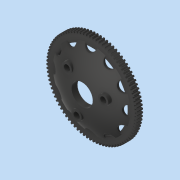
# Autodesk Inventor part: SpurGearLarge
Saved by Autodesk Inventor 2017 (Build 210142000, 142)
## iProperties
Created: 2016-11-06
Part Number: SpurGearLarge
Material: ABS Plastic
Document SubType Name: Modeling
Designer: techn
Density: 1.06 g/cm^3
Appearance: Smooth - Black
Author: techn
Autodesk Inventor part; units mm, degrees
ref_plane "YZ Plane" through (0, 0, 0) normal (1, 0, 0) x (0, 1, 0)
ref_plane "XZ Plane" through (0, 0, 0) normal (0, 1, 0) x (-1, 0, 0)
ref_plane "XY Plane" through (0, 0, 0) normal (0, 0, 1) x (1, 0, 0)
sketch "Sketch5" plane through (0, 0, 0) normal (0, 0, 1) x (1, 0, 0)
  circle A0 centre (0, 0) radius 22.86
  circle A1 centre (0, 0) radius 18.415
  dimension "d23" = 45.72
  dimension "d24" = 36.83
  constraints: 2 centre point, 2 coincident
  measures "d23" diameter of A0
  measures "d24" diameter of A1
extrude "Extrusion5" add sketch "Sketch5" along normal blind 3.175
sketch "Sketch6" plane through (0, 0, 0) normal (1, 0, 0) x (0, 1, 0)
  line L0 (22.86, 3.175) -> (-22.86, 3.175)
  line L1 (-22.86, 0) -> (22.86, 0)
  line L2 (22.86, 3.175) -> (-22.86, 3.175)
  line L3 (0, 3.175) -> (5.461, 3.175)
  line L4 (5.461, 3.175) -> (5.461, 7.9375)
  line L5 (22.86, 3.175) -> (19.685, 3.175)
  arc A0 (19.685, 3.175) -> (5.461, 7.9375) centre (0.085817, -31.738803) ccw
  line L6 (0, 3.175) -> (0, 13.966627)
  line L7 (-18.415, 3.175) -> (18.415, 3.175)
  line L8 (19.685, 3.175) -> (18.415, 3.175)
  arc A1 (18.415, 3.175) -> (5.461, 5.715) centre (1.432553, -49.132779) ccw
  point P0 (0, 0)
  dimension "d27" = 5.461
  dimension "d28" = 4.7625
  dimension "d29" = 3.175
  dimension "d36" = 2.54
  constraints: 10 end point, 4 point on circle, 3 point on line, 2 centre point, 1 horizontal, 1 midpoint, 1 perpendicular, 1 vertical
  measures "d27" distance of L3.start L3.end
  measures "d28" distance of L3.end L4.end
  measures "d29" distance of L0.start L5.end
  measures "d36" distance of L3.end A1.end
revolve "Revolution3" add sketch "Sketch6" angle 360 about axis through (0, 0, 3.175) along (0, 0, 1) contours L0 A1 L4 A0
sketch "Sketch8" plane through (0, 0, 3.175) normal (0, 0, 1) x (1, 0, 0)
  circle A0 centre (0, 0) radius 19.685
  circle A1 centre (0, 19.685) radius 2.8575
  circle A2 centre (-9.8425, 17.04771) radius 2.8575
  circle A3 centre (-17.04771, 9.8425) radius 2.8575
  circle A4 centre (-19.685, 0) radius 2.8575
  circle A5 centre (-17.04771, -9.8425) radius 2.8575
  circle A6 centre (-9.8425, -17.04771) radius 2.8575
  circle A7 centre (0, -19.685) radius 2.8575
  circle A8 centre (9.8425, -17.04771) radius 2.8575
  circle A9 centre (17.04771, -9.8425) radius 2.8575
  circle A10 centre (19.685, 0) radius 2.8575
  circle A11 centre (17.04771, 9.8425) radius 2.8575
  circle A12 centre (9.8425, 17.04771) radius 2.8575
  dimension "d38" = 5.715
  dimension "d41" = 360
  constraints: 12 centre point, 1 vertical alignment, 26 other
  measures "d38" diameter of A1
extrude "Extrusion6" cut sketch "Sketch8" along normal blind 3.175 contours A0 A10 | A0 A10 | A11 A0 | A0 A11 | A9 A0 | A0 A9 | A12 A0 | A0 A12 | A8 A0 | A0 A8 | A1 A0 | A0 A1 | A7 A0 | A0 A7 | A2 A0 | A0 A2 | A6 A0 | A0 A6 | A3 A0 | A0 A3 | A5 A0 | A0 A5 | A4 A0 | A0 A4
ref_plane "Work Plane1" through (0, 0, 7.9375) normal (0, 0, 1) x (1, 0, 0)
sketch "Sketch9" plane through (0, 0, 7.9375) normal (0, 0, 1) x (1, 0, 0)
  line L0 (0, 0) -> (12.7, 0) construction
  circle A0 centre (-7.77713, 7.77713) radius 1.5875
  circle A1 centre (-7.77713, 7.77713) radius 2.54
  circle A2 centre (-2.846627, -10.623757) radius 2.54
  circle A3 centre (-2.846627, -10.623757) radius 1.5875
  circle A4 centre (10.623757, 2.846627) radius 2.54
  circle A5 centre (10.623757, 2.846627) radius 1.5875
  dimension "d48" = 3.175
  dimension "d49" = 5.08
  dimension "d52" = 360
  dimension "d58" = 19.05
  constraints: 6 centre point, 3 coincident, 2 end point, 1 horizontal, 13 other
  measures "d48" diameter of A0
  measures "d49" diameter of A1
  measures "d58" distance of A4.centre A0.centre
extrude "Extrusion7" add sketch "Sketch9" against normal blind 2.286
extrude "Extrusion8" cut sketch "Sketch9" against normal through all contours A0 | A3 | A5
sketch "Sketch10" plane through (0, 0, 3.175) normal (0, 0, 1) x (1, 0, 0)
  circle A0 centre (0, 0) radius 21.8948
  line L0 (0.3683, 21.891702) -> (0.3683, 22.399702)
  line L1 (0.3683, 22.399702) -> (0.272875, 22.86)
  line L2 (0.272875, 22.86) -> (-0.272875, 22.86)
  line L3 (-0.272875, 22.86) -> (-0.3683, 22.399702)
  line L4 (-0.3683, 22.399702) -> (-0.3683, 21.891702)
  line L5 (-0.3683, 21.891702) -> (0.3683, 21.891702)
  line L6 (-1.983652, 22.314736) -> (-1.946996, 21.80806)
  line L7 (-1.92169, 22.780719) -> (-1.983652, 22.314736)
  line L8 (-1.377363, 22.820099) -> (-1.92169, 22.780719)
  line L9 (-1.248972, 22.367887) -> (-1.377363, 22.820099)
  line L10 (-1.212316, 21.861211) -> (-1.248972, 22.367887)
  line L11 (-1.946996, 21.80806) -> (-1.212316, 21.861211)
  line L12 (-3.588662, 22.11343) -> (-3.515541, 21.61072)
  line L13 (-3.560486, 22.58267) -> (-3.588662, 22.11343)
  line L14 (-3.02042, 22.661225) -> (-3.560486, 22.58267)
  line L15 (-2.859733, 22.219456) -> (-3.02042, 22.661225)
  line L16 (-2.786612, 21.716746) -> (-2.859733, 22.219456)
  line L17 (-3.515541, 21.61072) -> (-2.786612, 21.716746)
  line L18 (-5.174963, 21.796836) -> (-5.065758, 21.300713)
  line L19 (-5.180719, 22.266886) -> (-5.174963, 21.796836)
  line L20 (-4.647729, 22.384206) -> (-5.180719, 22.266886)
  line L21 (-4.455584, 21.955183) -> (-4.647729, 22.384206)
  line L22 (-4.346379, 21.45906) -> (-4.455584, 21.955183)
  line L23 (-5.065758, 21.300713) -> (-4.346379, 21.45906)
  line L24 (-6.734284, 21.366603) -> (-6.589565, 20.879653)
  line L25 (-6.773943, 21.835012) -> (-6.734284, 21.366603)
  line L26 (-6.250808, 21.990486) -> (-6.773943, 21.835012)
  line L27 (-6.028207, 21.576446) -> (-6.250808, 21.990486)
  line L28 (-5.883487, 21.089496) -> (-6.028207, 21.576446)
  line L29 (-6.589565, 20.879653) -> (-5.883487, 21.089496)
  line L30 (-8.258495, 20.824974) -> (-8.079016, 20.349736)
  line L31 (-8.33185, 21.289301) -> (-8.258495, 20.824974)
  line L32 (-7.821297, 21.482117) -> (-8.33185, 21.289301)
  line L33 (-7.5694, 21.085219) -> (-7.821297, 21.482117)
  line L34 (-7.389921, 20.609981) -> (-7.5694, 21.085219)
  line L35 (-8.079016, 20.349736) -> (-7.389921, 20.609981)
  line L36 (-9.739651, 20.174774) -> (-9.526347, 19.713726)
  line L37 (-9.846319, 20.632597) -> (-9.739651, 20.174774)
  line L38 (-9.351011, 20.861751) -> (-9.846319, 20.632597)
  line L39 (-9.071131, 20.484064) -> (-9.351011, 20.861751)
  line L40 (-8.857827, 20.023016) -> (-9.071131, 20.484064)
  line L41 (-9.526347, 19.713726) -> (-8.857827, 20.023016)
  line L42 (-11.170028, 19.419392) -> (-10.924012, 18.974937)
  line L43 (-11.309454, 19.868324) -> (-11.170028, 19.419392)
  line L44 (-10.831972, 20.132621) -> (-11.309454, 19.868324)
  line L45 (-10.525569, 19.776115) -> (-10.831972, 20.132621)
  line L46 (-10.279553, 19.33166) -> (-10.525569, 19.776115)
  line L47 (-10.924012, 18.974937) -> (-10.279553, 19.33166)
  line L48 (-12.54217, 18.562766) -> (-12.264725, 18.137221)
  line L49 (-12.713627, 19.000467) -> (-12.54217, 18.562766)
  line L50 (-12.25646, 19.29853) -> (-12.713627, 19.000467)
  line L51 (-11.925131, 18.965061) -> (-12.25646, 19.29853)
  line L52 (-11.647685, 18.539517) -> (-11.925131, 18.965061)
  line L53 (-12.264725, 18.137221) -> (-11.647685, 18.539517)
  line L54 (-13.848923, 17.609362) -> (-13.541495, 17.204947)
  line L55 (-14.051516, 18.033551) -> (-13.848923, 17.609362)
  line L56 (-13.617049, 18.363824) -> (-14.051516, 18.033551)
  line L57 (-13.262521, 18.055133) -> (-13.617049, 18.363824)
  line L58 (-12.955093, 17.650718) -> (-13.262521, 18.055133)
  line L59 (-13.541495, 17.204947) -> (-12.955093, 17.650718)
  line L60 (-15.083474, 16.564151) -> (-14.747666, 16.182973)
  line L61 (-15.316148, 16.972616) -> (-15.083474, 16.564151)
  line L62 (-14.906645, 17.333378) -> (-15.316148, 16.972616)
  line L63 (-14.530767, 17.051074) -> (-14.906645, 17.333378)
  line L64 (-14.194958, 16.669896) -> (-14.530767, 17.051074)
  line L65 (-14.747666, 16.182973) -> (-14.194958, 16.669896)
  line L66 (-16.239387, 15.432583) -> (-15.876949, 15.07663)
  line L67 (-16.500928, 15.823193) -> (-16.239387, 15.432583)
  line L68 (-16.118524, 16.212564) -> (-16.500928, 15.823193)
  line L69 (-15.723256, 15.958118) -> (-16.118524, 16.212564)
  line L70 (-15.360817, 15.602165) -> (-15.723256, 15.958118)
  line L71 (-15.876949, 15.07663) -> (-15.360817, 15.602165)
  line L72 (-17.310635, 14.220556) -> (-16.923457, 13.891683)
  line L73 (-17.59968, 14.591276) -> (-17.310635, 14.220556)
  line L74 (-17.246369, 15.007225) -> (-17.59968, 14.591276)
  line L75 (-16.833771, 14.781964) -> (-17.246369, 15.007225)
  line L76 (-16.446592, 14.453092) -> (-16.833771, 14.781964)
  line L77 (-16.923457, 13.891683) -> (-16.446592, 14.453092)
  line L78 (-18.291634, 12.934389) -> (-17.881734, 12.634312)
  line L79 (-18.606675, 13.283286) -> (-18.291634, 12.934389)
  line L80 (-18.2843, 13.723646) -> (-18.606675, 13.283286)
  line L81 (-17.856522, 13.528744) -> (-18.2843, 13.723646)
  line L82 (-17.446623, 13.228667) -> (-17.856522, 13.528744)
  line L83 (-17.881734, 12.634312) -> (-17.446623, 13.228667)
  line L84 (-19.177268, 11.580789) -> (-18.746784, 11.311072)
  line L85 (-19.516664, 11.906044) -> (-19.177268, 11.580789)
  line L86 (-19.226904, 12.368517) -> (-19.516664, 11.906044)
  line L87 (-18.786178, 12.204991) -> (-19.226904, 12.368517)
  line L88 (-18.355694, 11.935274) -> (-18.786178, 12.204991)
  line L89 (-18.746784, 11.311072) -> (-18.355694, 11.935274)
  line L90 (-19.962921, 10.166812) -> (-19.514097, 9.928861)
  line L91 (-20.324902, 10.466729) -> (-19.962921, 10.166812)
  line L92 (-20.069269, 10.948905) -> (-20.324902, 10.466729)
  line L93 (-19.617892, 10.817607) -> (-20.069269, 10.948905)
  line L94 (-19.169068, 10.579656) -> (-19.617892, 10.817607)
  line L95 (-19.514097, 9.928861) -> (-19.169068, 10.579656)
  line L96 (-20.644497, 8.69983) -> (-20.179673, 8.494885)
  line L97 (-21.027175, 8.972845) -> (-20.644497, 8.69983)
  line L98 (-20.807001, 9.47221) -> (-21.027175, 8.972845)
  line L99 (-20.347327, 9.373825) -> (-20.807001, 9.47221)
  line L100 (-19.882503, 9.16888) -> (-20.347327, 9.373825)
  line L101 (-20.179673, 8.494885) -> (-19.882503, 9.16888)
  line L102 (-21.218442, 7.187491) -> (-20.740041, 7.016621)
  line L103 (-21.619823, 7.432181) -> (-21.218442, 7.187491)
  line L104 (-21.436255, 7.946132) -> (-21.619823, 7.432181)
  line L105 (-20.97068, 7.881172) -> (-21.436255, 7.946132)
  line L106 (-20.492279, 7.710302) -> (-20.97068, 7.881172)
  line L107 (-20.740041, 7.016621) -> (-20.492279, 7.710302)
  line L108 (-21.681764, 5.63768) -> (-21.19228, 5.501775)
  line L109 (-22.099755, 5.852769) -> (-21.681764, 5.63768)
  line L110 (-21.953751, 6.378626) -> (-22.099755, 5.852769)
  line L111 (-21.484702, 6.347431) -> (-21.953751, 6.378626)
  line L112 (-20.995219, 6.211526) -> (-21.484702, 6.347431)
  line L113 (-21.19228, 5.501775) -> (-20.995219, 6.211526)
  line L114 (-22.032046, 4.058476) -> (-21.534032, 3.958246)
  line L115 (-22.464468, 4.242844) -> (-22.032046, 4.058476)
  line L116 (-22.35679, 4.777865) -> (-22.464468, 4.242844)
  line L117 (-21.886713, 4.780596) -> (-22.35679, 4.777865)
  line L118 (-21.388699, 4.680366) -> (-21.886713, 4.780596)
  line L119 (-21.534032, 3.958246) -> (-21.388699, 4.680366)
  line L120 (-22.267465, 2.458114) -> (-21.763516, 2.39408)
  line L121 (-22.712063, 2.610798) -> (-22.267465, 2.458114)
  line L122 (-22.643271, 3.152195) -> (-22.712063, 2.610798)
  line L123 (-22.174616, 3.188838) -> (-22.643271, 3.152195)
  line L124 (-21.670668, 3.124805) -> (-22.174616, 3.188838)
  line L125 (-21.763516, 2.39408) -> (-21.670668, 3.124805)
  line L126 (-22.38679, 0.844936) -> (-21.879535, 0.817433)
  line L127 (-22.841247, 0.965141) -> (-22.38679, 0.844936)
  line L128 (-22.811701, 1.51009) -> (-22.841247, 0.965141)
  line L129 (-22.346912, 1.580455) -> (-22.811701, 1.51009)
  line L130 (-21.839657, 1.552953) -> (-22.346912, 1.580455)
  line L131 (-21.879535, 0.817433) -> (-21.839657, 1.552953)
  line L132 (-22.389402, -0.772648) -> (-21.881485, -0.763476)
  line L133 (-22.851348, -0.685548) -> (-22.389402, -0.772648)
  line L134 (-22.861201, -0.139888) -> (-22.851348, -0.685548)
  line L135 (-22.402701, -0.036168) -> (-22.861201, -0.139888)
  line L136 (-21.894783, -0.026996) -> (-22.402701, -0.036168)
  line L137 (-21.881485, -0.763476) -> (-21.894783, -0.026996)
  line L138 (-22.275285, -2.386202) -> (-21.769354, -2.340405)
  line L139 (-22.742312, -2.332663) -> (-22.275285, -2.386202)
  line L140 (-22.791513, -1.789136) -> (-22.742312, -2.332663)
  line L141 (-22.341692, -1.652602) -> (-22.791513, -1.789136)
  line L142 (-21.835761, -1.606804) -> (-22.341692, -1.652602)
  line L143 (-21.769354, -2.340405) -> (-21.835761, -1.606804)
  line L144 (-22.045036, -3.987317) -> (-21.543728, -3.905131)
  line L145 (-22.514708, -3.967616) -> (-22.045036, -3.987317)
  line L146 (-22.603001, -3.429056) -> (-22.514708, -3.967616)
  line L147 (-22.164204, -3.26042) -> (-22.603001, -3.429056)
  line L148 (-21.662897, -3.178235) -> (-22.164204, -3.26042)
  line L149 (-21.543728, -3.905131) -> (-21.662897, -3.178235)
  line L150 (-21.699854, -5.567643) -> (-21.205783, -5.449499)
  line L151 (-22.169723, -5.581885) -> (-21.699854, -5.567643)
  line L152 (-22.296647, -5.0511) -> (-22.169723, -5.581885)
  line L153 (-21.871163, -4.85124) -> (-22.296647, -5.0511)
  line L154 (-21.377092, -4.733096) -> (-21.871163, -4.85124)
  line L155 (-21.205783, -5.449499) -> (-21.377092, -4.733096)
  line L156 (-21.241539, -7.118942) -> (-20.757281, -6.965455)
  line L157 (-21.709156, -7.167051) -> (-21.241539, -7.118942)
  line L158 (-21.874048, -6.646808) -> (-21.709156, -7.167051)
  line L159 (-21.464095, -6.416768) -> (-21.874048, -6.646808)
  line L160 (-20.979837, -6.263281) -> (-21.464095, -6.416768)
  line L161 (-20.757281, -6.965455) -> (-20.979837, -6.263281)
  line L162 (-20.67248, -8.633127) -> (-20.20056, -8.445096)
  line L163 (-21.135406, -8.714852) -> (-20.67248, -8.633127)
  line L164 (-21.337409, -8.207864) -> (-21.135406, -8.714852)
  line L165 (-20.945124, -7.948842) -> (-21.337409, -8.207864)
  line L166 (-20.473204, -7.760812) -> (-20.945124, -7.948842)
  line L167 (-20.20056, -8.445096) -> (-20.473204, -7.760812)
  line L168 (-19.995645, -10.102302) -> (-19.538522, -9.880709)
  line L169 (-20.451467, -10.217218) -> (-19.995645, -10.102302)
  line L170 (-20.689526, -9.726128) -> (-20.451467, -10.217218)
  line L171 (-20.316954, -9.439475) -> (-20.689526, -9.726128)
  line L172 (-19.859832, -9.217882) -> (-20.316954, -9.439475)
  line L173 (-19.538522, -9.880709) -> (-19.859832, -9.217882)
  line L174 (-19.214561, -11.518808) -> (-18.77462, -11.264808)
  line L175 (-19.660903, -11.666316) -> (-19.214561, -11.518808)
  line L176 (-19.933778, -11.193684) -> (-19.660903, -11.666316)
  line L177 (-19.582861, -10.880894) -> (-19.933778, -11.193684)
  line L178 (-19.14292, -10.626894) -> (-19.582861, -10.880894)
  line L179 (-18.77462, -11.264808) -> (-19.14292, -10.626894)
  line L180 (-18.333302, -12.875261) -> (-17.912836, -12.590178)
  line L181 (-18.767837, -13.054592) -> (-18.333302, -12.875261)
  line L182 (-19.074104, -12.602881) -> (-18.767837, -13.054592)
  line L183 (-18.746672, -12.265585) -> (-19.074104, -12.602881)
  line L184 (-18.326206, -11.980502) -> (-18.746672, -12.265585)
  line L185 (-17.912836, -12.590178) -> (-18.326206, -11.980502)
  line L186 (-17.356461, -14.164588) -> (-16.957662, -13.849908)
  line L187 (-17.776923, -14.374806) -> (-17.356461, -14.164588)
  line L188 (-18.114987, -13.946373) -> (-17.776923, -14.374806)
  line L189 (-17.812747, -13.586329) -> (-18.114987, -13.946373)
  line L190 (-17.413948, -13.27165) -> (-17.812747, -13.586329)
  line L191 (-16.957662, -13.849908) -> (-17.413948, -13.27165)
  line L192 (-16.289132, -15.380068) -> (-15.914079, -15.037432)
  line L193 (-16.693329, -15.620077) -> (-16.289132, -15.380068)
  line L194 (-17.061426, -15.217155) -> (-16.693329, -15.620077)
  line L195 (-16.785954, -14.836241) -> (-17.061426, -15.217155)
  line L196 (-16.410901, -14.493605) -> (-16.785954, -14.836241)
  line L197 (-15.914079, -15.037432) -> (-16.410901, -14.493605)
  line L198 (-15.136879, -16.515362) -> (-14.787528, -16.146557)
  line L199 (-15.522704, -16.783913) -> (-15.136879, -16.515362)
  line L200 (-15.918915, -16.408601) -> (-15.522704, -16.783913)
  line L201 (-15.671647, -16.008803) -> (-15.918915, -16.408601)
  line L202 (-15.322296, -15.639997) -> (-15.671647, -16.008803)
  line L203 (-14.787528, -16.146557) -> (-15.322296, -15.639997)
  line L204 (-13.905709, -17.564554) -> (-13.583881, -17.171501)
  line L205 (-14.27115, -17.860244) -> (-13.905709, -17.564554)
  line L206 (-14.693411, -17.514501) -> (-14.27115, -17.860244)
  line L207 (-14.475636, -17.097903) -> (-14.693411, -17.514501)
  line L208 (-14.153807, -16.70485) -> (-14.475636, -17.097903)
  line L209 (-13.583881, -17.171501) -> (-14.153807, -16.70485)
  line L210 (-12.602041, -18.522172) -> (-12.309414, -18.106921)
  line L211 (-12.945194, -18.843461) -> (-12.602041, -18.522172)
  line L212 (-13.391301, -18.529088) -> (-12.945194, -18.843461)
  line L213 (-13.204155, -18.097862) -> (-13.391301, -18.529088)
  line L214 (-12.911527, -17.682611) -> (-13.204155, -18.097862)
  line L215 (-12.309414, -18.106921) -> (-12.911527, -17.682611)
  line L216 (-11.232672, -19.383224) -> (-10.970771, -18.947941)
  line L217 (-11.551747, -19.728437) -> (-11.232672, -19.383224)
  line L218 (-12.019376, -19.447073) -> (-11.551747, -19.728437)
  line L219 (-11.863833, -19.003467) -> (-12.019376, -19.447073)
  line L220 (-11.601932, -18.568184) -> (-11.863833, -19.003467)
  line L221 (-10.970771, -18.947941) -> (-11.601932, -18.568184)
  line L222 (-9.804741, -20.143221) -> (-9.574932, -19.690174)
  line L223 (-10.098074, -20.510557) -> (-9.804741, -20.143221)
  line L224 (-10.584787, -20.263671) -> (-10.098074, -20.510557)
  line L225 (-10.46166, -19.809997) -> (-10.584787, -20.263671)
  line L226 (-10.23185, -19.35695) -> (-10.46166, -19.809997)
  line L227 (-9.574932, -19.690174) -> (-10.23185, -19.35695)
  line L228 (-8.325693, -20.7982) -> (-8.129173, -20.329752)
  line L229 (-8.591755, -21.185745) -> (-8.325693, -20.7982)
  line L230 (-9.095014, -20.974622) -> (-8.591755, -21.185745)
  line L231 (-9.004943, -20.513247) -> (-9.095014, -20.974622)
  line L232 (-8.808424, -20.044798) -> (-9.004943, -20.513247)
  line L233 (-8.129173, -20.329752) -> (-8.808424, -20.044798)
  line L234 (-6.803239, -21.344748) -> (-6.641033, -20.86334)
  line L235 (-7.040642, -21.750481) -> (-6.803239, -21.344748)
  line L236 (-7.557824, -21.576222) -> (-7.040642, -21.750481)
  line L237 (-7.50128, -21.10955) -> (-7.557824, -21.576222)
  line L238 (-7.339075, -20.628142) -> (-7.50128, -21.10955)
  line L239 (-6.641033, -20.86334) -> (-7.339075, -20.628142)
  line L240 (-5.245315, -21.780013) -> (-5.11827, -21.288156)
  line L241 (-5.452823, -22.201819) -> (-5.245315, -21.780013)
  line L242 (-5.98123, -22.065334) -> (-5.452823, -22.201819)
  line L243 (-5.958508, -21.595798) -> (-5.98123, -22.065334)
  line L244 (-5.831463, -21.103941) -> (-5.958508, -21.595798)
  line L245 (-5.11827, -21.288156) -> (-5.831463, -21.103941)
  line L246 (-3.660045, -22.101728) -> (-3.568822, -21.601985)
  line L247 (-3.836576, -22.537408) -> (-3.660045, -22.101728)
  line L248 (-4.373454, -22.439407) -> (-3.836576, -22.537408)
  line L249 (-4.384671, -21.969455) -> (-4.373454, -22.439407)
  line L250 (-4.293449, -21.469713) -> (-4.384671, -21.969455)
  line L251 (-3.568822, -21.601985) -> (-4.293449, -21.469713)
  line L252 (-2.055693, -22.308214) -> (-2.000768, -21.803192)
  line L253 (-2.200326, -22.755497) -> (-2.055693, -22.308214)
  line L254 (-2.742876, -22.696491) -> (-2.200326, -22.755497)
  line L255 (-2.787975, -22.228574) -> (-2.742876, -22.696491)
  line L256 (-2.73305, -21.723552) -> (-2.787975, -22.228574)
  line L257 (-2.000768, -21.803192) -> (-2.73305, -21.723552)
  line L258 (-0.440623, -22.398396) -> (-0.422283, -21.890727)
  line L259 (-0.552604, -22.854949) -> (-0.440623, -22.398396)
  line L260 (-1.097998, -22.835246) -> (-0.552604, -22.854949)
  line L261 (-1.176743, -22.371803) -> (-1.097998, -22.835246)
  line L262 (-1.158403, -21.864134) -> (-1.176743, -22.371803)
  line L263 (-0.422283, -21.890727) -> (-1.158403, -21.864134)
  line L264 (1.176743, -22.371803) -> (1.158403, -21.864134)
  line L265 (1.097998, -22.835246) -> (1.176743, -22.371803)
  line L266 (0.552604, -22.854949) -> (1.097998, -22.835246)
  line L267 (0.440623, -22.398396) -> (0.552604, -22.854949)
  line L268 (0.422283, -21.890727) -> (0.440623, -22.398396)
  line L269 (1.158403, -21.864134) -> (0.422283, -21.890727)
  line L270 (2.787975, -22.228574) -> (2.73305, -21.723552)
  line L271 (2.742876, -22.696491) -> (2.787975, -22.228574)
  line L272 (2.200326, -22.755497) -> (2.742876, -22.696491)
  line L273 (2.055693, -22.308214) -> (2.200326, -22.755497)
  line L274 (2.000768, -21.803192) -> (2.055693, -22.308214)
  line L275 (2.73305, -21.723552) -> (2.000768, -21.803192)
  line L276 (4.384671, -21.969455) -> (4.293449, -21.469713)
  line L277 (4.373454, -22.439407) -> (4.384671, -21.969455)
  line L278 (3.836576, -22.537408) -> (4.373454, -22.439407)
  line L279 (3.660045, -22.101728) -> (3.836576, -22.537408)
  line L280 (3.568822, -21.601985) -> (3.660045, -22.101728)
  line L281 (4.293449, -21.469713) -> (3.568822, -21.601985)
  line L282 (5.958508, -21.595798) -> (5.831463, -21.103941)
  line L283 (5.98123, -22.065334) -> (5.958508, -21.595798)
  line L284 (5.452823, -22.201819) -> (5.98123, -22.065334)
  line L285 (5.245315, -21.780013) -> (5.452823, -22.201819)
  line L286 (5.11827, -21.288156) -> (5.245315, -21.780013)
  line L287 (5.831463, -21.103941) -> (5.11827, -21.288156)
  line L288 (7.50128, -21.10955) -> (7.339075, -20.628142)
  line L289 (7.557824, -21.576222) -> (7.50128, -21.10955)
  line L290 (7.040642, -21.750481) -> (7.557824, -21.576222)
  line L291 (6.803239, -21.344748) -> (7.040642, -21.750481)
  line L292 (6.641033, -20.86334) -> (6.803239, -21.344748)
  line L293 (7.339075, -20.628142) -> (6.641033, -20.86334)
  line L294 (9.004943, -20.513247) -> (8.808424, -20.044798)
  line L295 (9.095014, -20.974622) -> (9.004943, -20.513247)
  line L296 (8.591755, -21.185745) -> (9.095014, -20.974622)
  line L297 (8.325693, -20.7982) -> (8.591755, -21.185745)
  line L298 (8.129173, -20.329752) -> (8.325693, -20.7982)
  line L299 (8.808424, -20.044798) -> (8.129173, -20.329752)
  line L300 (10.46166, -19.809997) -> (10.23185, -19.35695)
  line L301 (10.584787, -20.263671) -> (10.46166, -19.809997)
  line L302 (10.098074, -20.510557) -> (10.584787, -20.263671)
  line L303 (9.804741, -20.143221) -> (10.098074, -20.510557)
  line L304 (9.574932, -19.690174) -> (9.804741, -20.143221)
  line L305 (10.23185, -19.35695) -> (9.574932, -19.690174)
  line L306 (11.863833, -19.003467) -> (11.601932, -18.568184)
  line L307 (12.019376, -19.447073) -> (11.863833, -19.003467)
  line L308 (11.551747, -19.728437) -> (12.019376, -19.447073)
  line L309 (11.232672, -19.383224) -> (11.551747, -19.728437)
  line L310 (10.970771, -18.947941) -> (11.232672, -19.383224)
  line L311 (11.601932, -18.568184) -> (10.970771, -18.947941)
  line L312 (13.204155, -18.097862) -> (12.911527, -17.682611)
  line L313 (13.391301, -18.529088) -> (13.204155, -18.097862)
  line L314 (12.945194, -18.843461) -> (13.391301, -18.529088)
  line L315 (12.602041, -18.522172) -> (12.945194, -18.843461)
  line L316 (12.309414, -18.106921) -> (12.602041, -18.522172)
  line L317 (12.911527, -17.682611) -> (12.309414, -18.106921)
  line L318 (14.475636, -17.097903) -> (14.153807, -16.70485)
  line L319 (14.693411, -17.514501) -> (14.475636, -17.097903)
  line L320 (14.27115, -17.860244) -> (14.693411, -17.514501)
  line L321 (13.905709, -17.564554) -> (14.27115, -17.860244)
  line L322 (13.583881, -17.171501) -> (13.905709, -17.564554)
  line L323 (14.153807, -16.70485) -> (13.583881, -17.171501)
  line L324 (15.671647, -16.008803) -> (15.322296, -15.639997)
  line L325 (15.918915, -16.408601) -> (15.671647, -16.008803)
  line L326 (15.522704, -16.783913) -> (15.918915, -16.408601)
  line L327 (15.136879, -16.515362) -> (15.522704, -16.783913)
  line L328 (14.787528, -16.146557) -> (15.136879, -16.515362)
  line L329 (15.322296, -15.639997) -> (14.787528, -16.146557)
  line L330 (16.785954, -14.836241) -> (16.410901, -14.493605)
  line L331 (17.061426, -15.217155) -> (16.785954, -14.836241)
  line L332 (16.693329, -15.620077) -> (17.061426, -15.217155)
  line L333 (16.289132, -15.380068) -> (16.693329, -15.620077)
  line L334 (15.914079, -15.037432) -> (16.289132, -15.380068)
  line L335 (16.410901, -14.493605) -> (15.914079, -15.037432)
  line L336 (17.812747, -13.586329) -> (17.413948, -13.27165)
  line L337 (18.114987, -13.946373) -> (17.812747, -13.586329)
  line L338 (17.776923, -14.374806) -> (18.114987, -13.946373)
  line L339 (17.356461, -14.164588) -> (17.776923, -14.374806)
  line L340 (16.957662, -13.849908) -> (17.356461, -14.164588)
  line L341 (17.413948, -13.27165) -> (16.957662, -13.849908)
  line L342 (18.746672, -12.265585) -> (18.326206, -11.980502)
  line L343 (19.074104, -12.602881) -> (18.746672, -12.265585)
  line L344 (18.767837, -13.054592) -> (19.074104, -12.602881)
  line L345 (18.333302, -12.875261) -> (18.767837, -13.054592)
  line L346 (17.912836, -12.590178) -> (18.333302, -12.875261)
  line L347 (18.326206, -11.980502) -> (17.912836, -12.590178)
  line L348 (19.582861, -10.880894) -> (19.14292, -10.626894)
  line L349 (19.933778, -11.193684) -> (19.582861, -10.880894)
  line L350 (19.660903, -11.666316) -> (19.933778, -11.193684)
  line L351 (19.214561, -11.518808) -> (19.660903, -11.666316)
  line L352 (18.77462, -11.264808) -> (19.214561, -11.518808)
  line L353 (19.14292, -10.626894) -> (18.77462, -11.264808)
  line L354 (20.316954, -9.439475) -> (19.859832, -9.217882)
  line L355 (20.689526, -9.726128) -> (20.316954, -9.439475)
  line L356 (20.451467, -10.217218) -> (20.689526, -9.726128)
  line L357 (19.995645, -10.102302) -> (20.451467, -10.217218)
  line L358 (19.538522, -9.880709) -> (19.995645, -10.102302)
  line L359 (19.859832, -9.217882) -> (19.538522, -9.880709)
  line L360 (20.945124, -7.948842) -> (20.473204, -7.760812)
  line L361 (21.337409, -8.207864) -> (20.945124, -7.948842)
  line L362 (21.135406, -8.714852) -> (21.337409, -8.207864)
  line L363 (20.67248, -8.633127) -> (21.135406, -8.714852)
  line L364 (20.20056, -8.445096) -> (20.67248, -8.633127)
  line L365 (20.473204, -7.760812) -> (20.20056, -8.445096)
  line L366 (21.464095, -6.416768) -> (20.979837, -6.263281)
  line L367 (21.874048, -6.646808) -> (21.464095, -6.416768)
  line L368 (21.709156, -7.167051) -> (21.874048, -6.646808)
  line L369 (21.241539, -7.118942) -> (21.709156, -7.167051)
  line L370 (20.757281, -6.965455) -> (21.241539, -7.118942)
  line L371 (20.979837, -6.263281) -> (20.757281, -6.965455)
  line L372 (21.871163, -4.85124) -> (21.377092, -4.733096)
  line L373 (22.296647, -5.0511) -> (21.871163, -4.85124)
  line L374 (22.169723, -5.581885) -> (22.296647, -5.0511)
  line L375 (21.699854, -5.567643) -> (22.169723, -5.581885)
  line L376 (21.205783, -5.449499) -> (21.699854, -5.567643)
  line L377 (21.377092, -4.733096) -> (21.205783, -5.449499)
  line L378 (22.164204, -3.26042) -> (21.662897, -3.178235)
  line L379 (22.603001, -3.429056) -> (22.164204, -3.26042)
  line L380 (22.514708, -3.967616) -> (22.603001, -3.429056)
  line L381 (22.045036, -3.987317) -> (22.514708, -3.967616)
  line L382 (21.543728, -3.905131) -> (22.045036, -3.987317)
  line L383 (21.662897, -3.178235) -> (21.543728, -3.905131)
  line L384 (22.341692, -1.652602) -> (21.835761, -1.606804)
  line L385 (22.791513, -1.789136) -> (22.341692, -1.652602)
  line L386 (22.742312, -2.332663) -> (22.791513, -1.789136)
  line L387 (22.275285, -2.386202) -> (22.742312, -2.332663)
  line L388 (21.769354, -2.340405) -> (22.275285, -2.386202)
  line L389 (21.835761, -1.606804) -> (21.769354, -2.340405)
  line L390 (22.402701, -0.036168) -> (21.894783, -0.026996)
  line L391 (22.861201, -0.139888) -> (22.402701, -0.036168)
  line L392 (22.851348, -0.685548) -> (22.861201, -0.139888)
  line L393 (22.389402, -0.772648) -> (22.851348, -0.685548)
  line L394 (21.881485, -0.763476) -> (22.389402, -0.772648)
  line L395 (21.894783, -0.026996) -> (21.881485, -0.763476)
  line L396 (22.346912, 1.580455) -> (21.839657, 1.552953)
  line L397 (22.811701, 1.51009) -> (22.346912, 1.580455)
  line L398 (22.841247, 0.965141) -> (22.811701, 1.51009)
  line L399 (22.38679, 0.844936) -> (22.841247, 0.965141)
  line L400 (21.879535, 0.817433) -> (22.38679, 0.844936)
  line L401 (21.839657, 1.552953) -> (21.879535, 0.817433)
  line L402 (22.174616, 3.188838) -> (21.670668, 3.124805)
  line L403 (22.643271, 3.152195) -> (22.174616, 3.188838)
  line L404 (22.712063, 2.610798) -> (22.643271, 3.152195)
  line L405 (22.267465, 2.458114) -> (22.712063, 2.610798)
  line L406 (21.763516, 2.39408) -> (22.267465, 2.458114)
  line L407 (21.670668, 3.124805) -> (21.763516, 2.39408)
  line L408 (21.886713, 4.780596) -> (21.388699, 4.680366)
  line L409 (22.35679, 4.777865) -> (21.886713, 4.780596)
  line L410 (22.464468, 4.242844) -> (22.35679, 4.777865)
  line L411 (22.032046, 4.058476) -> (22.464468, 4.242844)
  line L412 (21.534032, 3.958246) -> (22.032046, 4.058476)
  line L413 (21.388699, 4.680366) -> (21.534032, 3.958246)
  line L414 (21.484702, 6.347431) -> (20.995219, 6.211526)
  line L415 (21.953751, 6.378626) -> (21.484702, 6.347431)
  line L416 (22.099755, 5.852769) -> (21.953751, 6.378626)
  line L417 (21.681764, 5.63768) -> (22.099755, 5.852769)
  line L418 (21.19228, 5.501775) -> (21.681764, 5.63768)
  line L419 (20.995219, 6.211526) -> (21.19228, 5.501775)
  line L420 (20.97068, 7.881172) -> (20.492279, 7.710302)
  line L421 (21.436255, 7.946132) -> (20.97068, 7.881172)
  line L422 (21.619823, 7.432181) -> (21.436255, 7.946132)
  line L423 (21.218442, 7.187491) -> (21.619823, 7.432181)
  line L424 (20.740041, 7.016621) -> (21.218442, 7.187491)
  line L425 (20.492279, 7.710302) -> (20.740041, 7.016621)
  line L426 (20.347327, 9.373825) -> (19.882503, 9.16888)
  line L427 (20.807001, 9.47221) -> (20.347327, 9.373825)
  line L428 (21.027175, 8.972845) -> (20.807001, 9.47221)
  line L429 (20.644497, 8.69983) -> (21.027175, 8.972845)
  line L430 (20.179673, 8.494885) -> (20.644497, 8.69983)
  line L431 (19.882503, 9.16888) -> (20.179673, 8.494885)
  line L432 (19.617892, 10.817607) -> (19.169068, 10.579656)
  line L433 (20.069269, 10.948905) -> (19.617892, 10.817607)
  line L434 (20.324902, 10.466729) -> (20.069269, 10.948905)
  line L435 (19.962921, 10.166812) -> (20.324902, 10.466729)
  line L436 (19.514097, 9.928861) -> (19.962921, 10.166812)
  line L437 (19.169068, 10.579656) -> (19.514097, 9.928861)
  line L438 (18.786178, 12.204991) -> (18.355694, 11.935274)
  line L439 (19.226904, 12.368517) -> (18.786178, 12.204991)
  line L440 (19.516664, 11.906044) -> (19.226904, 12.368517)
  line L441 (19.177268, 11.580789) -> (19.516664, 11.906044)
  line L442 (18.746784, 11.311072) -> (19.177268, 11.580789)
  line L443 (18.355694, 11.935274) -> (18.746784, 11.311072)
  line L444 (17.856522, 13.528744) -> (17.446623, 13.228667)
  line L445 (18.2843, 13.723646) -> (17.856522, 13.528744)
  line L446 (18.606675, 13.283286) -> (18.2843, 13.723646)
  line L447 (18.291634, 12.934389) -> (18.606675, 13.283286)
  line L448 (17.881734, 12.634312) -> (18.291634, 12.934389)
  line L449 (17.446623, 13.228667) -> (17.881734, 12.634312)
  line L450 (16.833771, 14.781964) -> (16.446592, 14.453092)
  line L451 (17.246369, 15.007225) -> (16.833771, 14.781964)
  line L452 (17.59968, 14.591276) -> (17.246369, 15.007225)
  line L453 (17.310635, 14.220556) -> (17.59968, 14.591276)
  line L454 (16.923457, 13.891683) -> (17.310635, 14.220556)
  line L455 (16.446592, 14.453092) -> (16.923457, 13.891683)
  line L456 (15.723256, 15.958118) -> (15.360817, 15.602165)
  line L457 (16.118524, 16.212564) -> (15.723256, 15.958118)
  line L458 (16.500928, 15.823193) -> (16.118524, 16.212564)
  line L459 (16.239387, 15.432583) -> (16.500928, 15.823193)
  line L460 (15.876949, 15.07663) -> (16.239387, 15.432583)
  line L461 (15.360817, 15.602165) -> (15.876949, 15.07663)
  line L462 (14.530767, 17.051074) -> (14.194958, 16.669896)
  line L463 (14.906645, 17.333378) -> (14.530767, 17.051074)
  line L464 (15.316148, 16.972616) -> (14.906645, 17.333378)
  line L465 (15.083474, 16.564151) -> (15.316148, 16.972616)
  line L466 (14.747666, 16.182973) -> (15.083474, 16.564151)
  line L467 (14.194958, 16.669896) -> (14.747666, 16.182973)
  line L468 (13.262521, 18.055133) -> (12.955093, 17.650718)
  line L469 (13.617049, 18.363824) -> (13.262521, 18.055133)
  line L470 (14.051516, 18.033551) -> (13.617049, 18.363824)
  line L471 (13.848923, 17.609362) -> (14.051516, 18.033551)
  line L472 (13.541495, 17.204947) -> (13.848923, 17.609362)
  line L473 (12.955093, 17.650718) -> (13.541495, 17.204947)
  line L474 (11.925131, 18.965061) -> (11.647685, 18.539517)
  line L475 (12.25646, 19.29853) -> (11.925131, 18.965061)
  line L476 (12.713627, 19.000467) -> (12.25646, 19.29853)
  line L477 (12.54217, 18.562766) -> (12.713627, 19.000467)
  line L478 (12.264725, 18.137221) -> (12.54217, 18.562766)
  line L479 (11.647685, 18.539517) -> (12.264725, 18.137221)
  line L480 (10.525569, 19.776115) -> (10.279553, 19.33166)
  line L481 (10.831972, 20.132621) -> (10.525569, 19.776115)
  line L482 (11.309454, 19.868324) -> (10.831972, 20.132621)
  line L483 (11.170028, 19.419392) -> (11.309454, 19.868324)
  line L484 (10.924012, 18.974937) -> (11.170028, 19.419392)
  line L485 (10.279553, 19.33166) -> (10.924012, 18.974937)
  line L486 (9.071131, 20.484064) -> (8.857827, 20.023016)
  line L487 (9.351011, 20.861751) -> (9.071131, 20.484064)
  line L488 (9.846319, 20.632597) -> (9.351011, 20.861751)
  line L489 (9.739651, 20.174774) -> (9.846319, 20.632597)
  line L490 (9.526347, 19.713726) -> (9.739651, 20.174774)
  line L491 (8.857827, 20.023016) -> (9.526347, 19.713726)
  line L492 (7.5694, 21.085219) -> (7.389921, 20.609981)
  line L493 (7.821297, 21.482117) -> (7.5694, 21.085219)
  line L494 (8.33185, 21.289301) -> (7.821297, 21.482117)
  line L495 (8.258495, 20.824974) -> (8.33185, 21.289301)
  line L496 (8.079016, 20.349736) -> (8.258495, 20.824974)
  line L497 (7.389921, 20.609981) -> (8.079016, 20.349736)
  line L498 (6.028207, 21.576446) -> (5.883487, 21.089496)
  line L499 (6.250808, 21.990486) -> (6.028207, 21.576446)
  line L500 (6.773943, 21.835012) -> (6.250808, 21.990486)
  line L501 (6.734284, 21.366603) -> (6.773943, 21.835012)
  line L502 (6.589565, 20.879653) -> (6.734284, 21.366603)
  line L503 (5.883487, 21.089496) -> (6.589565, 20.879653)
  line L504 (4.455584, 21.955183) -> (4.346379, 21.45906)
  line L505 (4.647729, 22.384206) -> (4.455584, 21.955183)
  line L506 (5.180719, 22.266886) -> (4.647729, 22.384206)
  line L507 (5.174963, 21.796836) -> (5.180719, 22.266886)
  line L508 (5.065758, 21.300713) -> (5.174963, 21.796836)
  line L509 (4.346379, 21.45906) -> (5.065758, 21.300713)
  line L510 (2.859733, 22.219456) -> (2.786612, 21.716746)
  line L511 (3.02042, 22.661225) -> (2.859733, 22.219456)
  line L512 (3.560486, 22.58267) -> (3.02042, 22.661225)
  line L513 (3.588662, 22.11343) -> (3.560486, 22.58267)
  line L514 (3.515541, 21.61072) -> (3.588662, 22.11343)
  line L515 (2.786612, 21.716746) -> (3.515541, 21.61072)
  line L516 (1.248972, 22.367887) -> (1.212316, 21.861211)
  line L517 (1.377363, 22.820099) -> (1.248972, 22.367887)
  line L518 (1.92169, 22.780719) -> (1.377363, 22.820099)
  line L519 (1.983652, 22.314736) -> (1.92169, 22.780719)
  line L520 (1.946996, 21.80806) -> (1.983652, 22.314736)
  line L521 (1.212316, 21.861211) -> (1.946996, 21.80806)
  circle A1 centre (0, 0) radius 25.183748
  dimension "d59" = 0.508
  dimension "d60" = 0.9652
  dimension "d61" = 0.7366
  dimension "d64" = 360
  constraints: 1044 end point, 2 centre point, 2 coincident, 2 equal length, 2 point on circle, 1 horizontal, 1 parallel, 1 perpendicular, 1 vertical, 1045 other
  measures "d59" distance of L0.start L0.end
  measures "d60" distance edge to line of A0 L2
  measures "d61" distance between parallel lines of L0 L4
extrude "Extrusion9" cut sketch "Sketch10" against normal through all
ref_plane "Work Plane2" through (0, 0, 5.715) normal (0, 0, -1) x (-1, 0, 0)
sketch "Sketch11" plane through (0, 0, 5.715) normal (0, 0, -1) x (-1, 0, 0)
  spline S0 degree 2 poles (-12.211257, 2.846627) (-12.211257, 5.596258) (-9.830007, 4.221442) (-7.448757, 2.846627) (-9.830007, 1.471812) (-12.211257, 0.096996) (-12.211257, 2.846627) knots 0 0 0 0.33333333 0.33333333 0.66666667 0.66666667 1 1 1 weights 1 0.5 1 0.5 1 0.5 1
  spline S1 degree 2 poles (6.18963, 7.77713) (6.18963, 10.526761) (8.57088, 9.151945) (10.95213, 7.77713) (8.57088, 6.402315) (6.18963, 5.027499) (6.18963, 7.77713) knots 0 0 0 0.33333333 0.33333333 0.66666667 0.66666667 1 1 1 weights 1 0.5 1 0.5 1 0.5 1
  spline S2 degree 2 poles (1.259127, -10.623757) (1.259127, -7.874126) (3.640377, -9.248942) (6.021627, -10.623757) (3.640377, -11.998572) (1.259127, -13.373388) (1.259127, -10.623757) knots 0 0 0 0.33333333 0.33333333 0.66666667 0.66666667 1 1 1 weights 1 0.5 1 0.5 1 0.5 1
  circle A0 centre (0, 0) radius 11.43
  circle A1 centre (0, 0) radius 5.461
  dimension "d69" = 22.86
  constraints: 1 centre point, 1 coincident, 3 other
  measures "d69" diameter of A0
extrude "Extrusion10" add sketch "Sketch11" along normal blind 0.7874 contours A0 S1 S2 S0 | S0 A0 | A0 S1 | S2 A0 picked at (-10.382403, 2.783832) picked at (7.62267, 7.580116) picked at (2.830527, -10.372293)
extrude "Extrusion11" cut sketch "Sketch11" along normal through all contours S0 A0 | S0 A0 | A0 S1 | S1 A0 | A0 S2 | S2 A0
body "Solid2"
